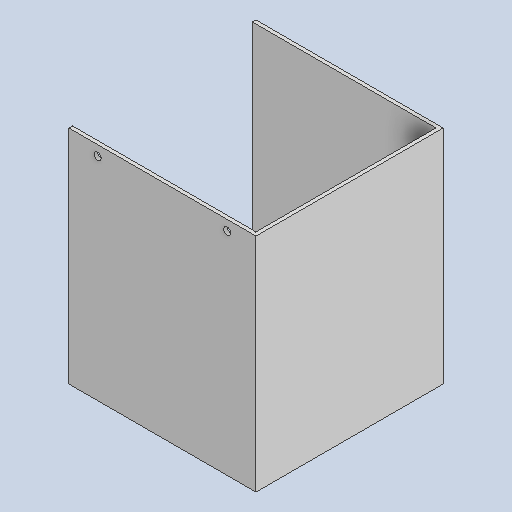
# Autodesk Inventor part: Low
Saved by Autodesk Inventor 2025 (Build 290162000, 162)
## iProperties
Created: 2025-08-07
Part Number: Low
Material: Generic
Document SubType Name: Modeling
Designer: Pravoslav
Density: 1 g/cm^3
Appearance: Default
Author: Pravoslav
Autodesk Inventor part; units mm, degrees
ref_plane "YZ Plane" through (0, 0, 0) normal (1, 0, 0) x (0, 1, 0)
ref_plane "XZ Plane" through (0, 0, 0) normal (0, 1, 0) x (-1, 0, 0)
ref_plane "XY Plane" through (0, 0, 0) normal (0, 0, 1) x (1, 0, 0)
sketch "Sketch1" plane through (0, 0, 0) normal (0, 1, 0) x (-1, 0, 0)
  line L0 (65, 65) -> (-65, 65)
  line L1 (-65, 65) -> (-65, -65)
  line L2 (-65, -65) -> (65, -65)
  line L3 (65, -65) -> (65, 65)
  line L4 (65, 65) -> (-65, -65) construction
  line L5 (-65, 65) -> (65, -65) construction
  line L6 (55.5, 55.5) -> (-55.5, 55.5)
  line L7 (-55.5, 55.5) -> (-55.5, -55.5)
  line L8 (-55.5, -55.5) -> (55.5, -55.5)
  line L9 (55.5, -55.5) -> (55.5, 55.5)
  line L10 (55.5, 55.5) -> (-55.5, -55.5) construction
  line L11 (-55.5, 55.5) -> (55.5, -55.5) construction
  circle A0 centre (55.5, 55.5) radius 2.5
  circle A1 centre (55.5, -55.5) radius 2.5
  circle A2 centre (-55.5, -55.5) radius 2.5
  circle A3 centre (-55.5, 55.5) radius 2.5
  point P0 (0, 0)
  dimension "d0" = 130
  dimension "d1" = 130
  dimension "d2" = 111
  dimension "d3" = 5
  dimension "d4" = 5
  dimension "d5" = 5
  dimension "d6" = 5
  constraints: 24 end point, 4 centre point, 4 midpoint, 4 parallel, 3 coincident, 2 horizontal, 2 perpendicular, 2 point on line
  measures "d0" distance of L2.end L1.end
  measures "d1" distance of L1.end L0.end
  measures "d2" distance of L8.end L7.end
  measures "d3" diameter of A0
  measures "d4" diameter of A1
  measures "d5" diameter of A2
  measures "d6" diameter of A3
extrude "Extrusion1" add sketch "Sketch1" along normal blind 4 contours L3 L2 L1 L0 | L6 A0 L9 A1 L8 A2 L7 A3
sketch "Sketch2" plane through (0, 4, 0) normal (0, 1, 0) x (1, 0, 0)
  line L0 (-62.5, -62.5) -> (62.5, -62.5)
  line L1 (62.5, -62.5) -> (62.5, 62.5)
  line L2 (62.5, 62.5) -> (-62.5, 62.5)
  line L3 (-62.5, 62.5) -> (-62.5, -62.5)
  line L4 (-62.5, -62.5) -> (62.5, 62.5) construction
  line L5 (62.5, -62.5) -> (-62.5, 62.5) construction
  line L6 (65, -65) -> (65, 65) projected
  line L7 (-65, -65) -> (65, -65)
  line L8 (65, -65) -> (65, 65)
  line L9 (65, 65) -> (-65, 65)
  line L10 (-65, 65) -> (-65, -65)
  line L11 (-65, -65) -> (65, 65) construction
  line L12 (65, -65) -> (-65, 65) construction
  line L13 (-62.5, -62.5) -> (-65, -62.5)
  line L14 (-62.5, 62.5) -> (-65, 62.5)
  point P0 (0, 0)
  dimension "d9" = 125
  dimension "d10" = 125
  constraints: 28 end point, 4 midpoint, 4 parallel, 4 perpendicular, 2 horizontal, 2 point on line
  measures "d9" distance of L2.end L1.end
  measures "d10" distance of L1.end L0.end
extrude "Extrusion2" add sketch "Sketch2" along normal blind 150 contours L0 L1 L2 L14 L10 L9 L6 L7 L13
sketch "Sketch3" plane through (-65, 0, 65) normal (0, 0, 1) x (1, 0, 0)
  circle A0 centre (20, 147) radius 2.5
  circle A1 centre (110, 147) radius 2.5
  line L0 (0, 154) -> (130, 154) projected
  line L1 (130, 0) -> (130, 154) projected
  line L2 (0, 0) -> (0, 154) projected
  point P0 (65, 0)
  dimension "d13" = 5
  dimension "d14" = 5
  dimension "d15" = 7
  dimension "d16" = 7
  dimension "d17" = 20
  dimension "d18" = 20
  constraints: 2 centre point
  measures "d13" diameter of A0
  measures "d14" diameter of A1
  measures "d15" distance from line of L0 A0.centre
  measures "d16" distance from line of L0 A1.centre
  measures "d17" distance from line of L1 A1.centre
  measures "d18" distance from line of L2 A0.centre
extrude "Extrusion3" cut sketch "Sketch3" against normal up to surface (2.5 mm away)
body "Solid1"
